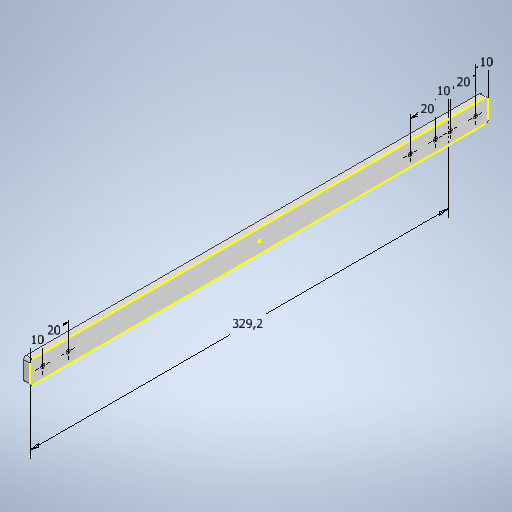
# Autodesk Inventor part: Sstab
Saved by Autodesk Inventor 2025.1 (Build 291241000, 241)
## iProperties
Created: 2024-11-26
Part Number: Sstab
Material: Generisch
Document SubType Name: Modeling
Designer: Kai Altwicker
Density: 1 g/cm^3
Appearance: Vorgabe
Author: Kai Altwicker
Autodesk Inventor part; units mm, degrees
ref_plane "YZ Plane" through (0, 0, 0) normal (1, 0, 0) x (0, 1, 0)
ref_plane "XZ Plane" through (0, 0, 0) normal (0, 1, 0) x (-1, 0, 0)
ref_plane "XY Plane" through (0, 0, 0) normal (0, 0, 1) x (1, 0, 0)
sketch "Skizze1" plane through (0, 0, 0) normal (1, 0, 0) x (0, 1, 0)
  line L0 (9, 180.35) -> (-9, 180.35)
  line L1 (-9, 180.35) -> (-9, -180.35)
  line L2 (-9, -180.35) -> (9, -180.35)
  line L3 (9, -180.35) -> (9, 180.35)
  point P0 (0, 0)
  point P1 (-9, 0)
  point P2 (0, -180.35)
  dimension "d0" = 360.7
  dimension "d1" = 18
  constraints: 8 end point, 2 midpoint, 2 parallel, 1 horizontal, 1 horizontal alignment, 1 perpendicular, 1 vertical alignment
  measures "d0" distance of L0.end L1.end
  measures "d1" distance of L0.start L0.end
extrude "Extrusion1" add sketch "Skizze1" along normal blind 5
fillet "Rundung1" radius 2 4 edges at (2.5, 9, 180.35) (2.5, -9, 180.35) (2.5, 9, -180.35) (2.5, -9, -180.35)
sketch "Skizze2" plane through (5, 0, 0) normal (1, 0, 0) x (0, 0, -1)
  line L0 (-180.35, 7) -> (-180.35, -7) projected
  line L1 (178.35, 9) -> (-178.35, 9) projected
  line L2 (148.85, 9) -> (148.85, -9) construction
  line L3 (-178.35, -9) -> (178.35, -9) projected
  line L4 (180.35, -7) -> (180.35, 7) projected
  point P0 (0, 0)
  point P1 (-170.35, 0)
  point P2 (-150.35, 0)
  point P3 (138.85, 0)
  point P4 (118.85, 0)
  point P5 (170.35, 0)
  point P6 (150.35, 0)
  dimension "d5" = 10
  dimension "d6" = 20
  dimension "d7" = 329.2
  dimension "d8" = 10
  dimension "d9" = 20
  dimension "d10" = 10
  dimension "d11" = 20
  constraints: 6 horizontal alignment, 2 end point, 2 point on line
  measures "d5" distance from line of L0 point (-170.35, 0)
  measures "d6" distance of point (-170.35, 0) point (-150.35, 0)
  measures "d7" distance between parallel lines of L0 L2
  measures "d8" distance from line of L2 point (138.85, 0)
  measures "d9" distance of point (138.85, 0) point (118.85, 0)
  measures "d10" distance from line of L4 point (170.35, 0)
  measures "d11" distance of point (170.35, 0) point (150.35, 0)
hole "Bohrung1" at (5, 0, -138.85) at (5, 0, -118.85) at (5, 0, -170.35) at (5, 0, -150.35) at (5, 0, 150.35) at (5, 0, 170.35) direction (-1, 0, 0) diameter 3.242 end through all thread size "M4x0.7" class "6H" standard "ISO Metric profile"
equation "\"d_tol\" = 0.3"
equation "\"d_wand\" = 1.5"
equation "\"b_rasp_pi\" = 56"
equation "\"w_kamera_hori\" = 66deg"
equation "\"l_rasp_pi\" = 85"
equation "\"w_kamera_vert\" = 41deg"
equation "\"r_rasp_pi\" = 3"
equation "\"D_oct\" = 3621.32034"
equation "\"D_hexadeca\" = 7541.00924"
equation "\"d_traeger\" = 625"
